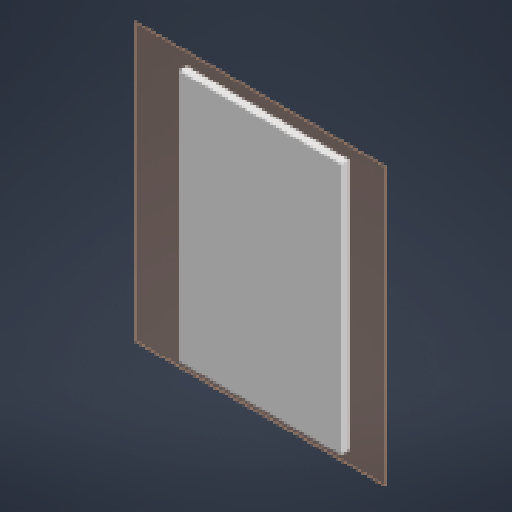
# Autodesk Inventor part: Szkło
Saved by Autodesk Inventor 2025 (Build 290162000, 162)
## iProperties
Created: 2024-04-15
Part Number: Szkło
Material: Generic
Document SubType Name: Modeling
Designer: sicia
Density: 1 g/cm^3
Appearance: Default
Author: sicia
Autodesk Inventor part; units mm, degrees
ref_plane "YZ Plane" through (0, 0, 0) normal (1, 0, 0) x (0, 1, 0)
ref_plane "XZ Plane" through (0, 0, 0) normal (0, 1, 0) x (-1, 0, 0)
ref_plane "XY Plane" through (0, 0, 0) normal (0, 0, 1) x (1, 0, 0)
ref_plane "Work Plane1" through (0, 0, 0) normal (0, 0, 1) x (1, 0, 0)
sketch "Sketch1" plane through (0, 0, 0) normal (0, 0, 1) x (1, 0, 0)
  arc A0 (28, 29) -> (26, 31) centre (26, 29) ccw projected
  line L0 (26, 31) -> (-26, 31) projected
  arc A1 (-26, 31) -> (-26, 27) centre (-26, 29) ccw projected
  line L1 (-26, 27) -> (-24, 27) projected
  line L2 (-24, 27) -> (-24, -27) projected
  line L3 (-24, -27) -> (-26, -27) projected
  arc A2 (-26, -27) -> (-26, -31) centre (-26, -29) ccw projected
  line L4 (-26, -31) -> (26, -31) projected
  arc A3 (26, -31) -> (28, -29) centre (26, -29) ccw projected
  line L5 (28, -29) -> (28, 29) projected
  line L6 (22, 31) -> (-18, 31)
  line L7 (-18, 31) -> (-18, -31)
  line L8 (-18, -31) -> (22, -31)
  line L9 (22, -31) -> (22, 31)
  point P0 (0, 0)
  point P1 (22, -31)
  point P2 (-18, -31)
  dimension "d0" = 40
  dimension "d1" = 62
  dimension "d2" = 6
  dimension "d3" = 0
  constraints: 8 end point, 2 parallel, 1 horizontal, 1 perpendicular
  measures "d0" distance of L8.end L7.end
  measures "d1" distance of L7.end L6.end
  measures "d2" distance between parallel lines of L5 L9
  measures "d3" distance between parallel lines of L0 L6
extrude "Extrusion1" add sketch "Sketch1" along normal blind 2 contours L9 L4 L7 L0
body "Solid1"
